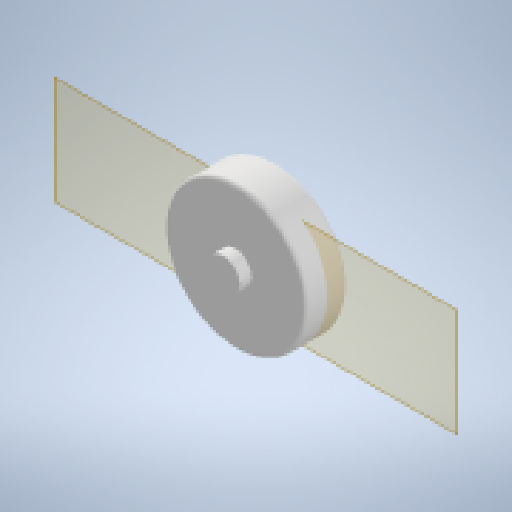
# Autodesk Inventor part: Колесо
Saved by Autodesk Inventor 2024.2 (Build 282272000, 272)
## iProperties
Created: 2025-03-03
Part Number: Колесо
Material: Типовые
Document SubType Name: Modeling
Designer: Timofey
Density: 1 g/cm^3
Appearance: По умолчанию
Mass: 1234.52 g
Surface Area: 769.826 cm^2
Volume: 1234.52 cm^3
Author: Timofey
Autodesk Inventor part; units mm, degrees
ref_plane "YZ Plane" through (0, 0, 0) normal (1, 0, 0) x (0, 1, 0)
ref_plane "XZ Plane" through (0, 0, 0) normal (0, 1, 0) x (-1, 0, 0)
ref_plane "XY Plane" through (0, 0, 0) normal (0, 0, 1) x (1, 0, 0)
ref_plane "РабПлоскость3" through (0.0801, 60, -30) normal (0, 0, 1) x (1, 0, 0)
sketch "Эскиз1" plane through (0.0801, 60, -30) normal (0, 0, 1) x (1, 0, 0)
  line L0 (-0.0801, -60) -> (-90.0801, -60)
  circle A0 centre (-90.0801, -60) radius 87.5
  dimension "d0" = 90
  dimension "d1" = 175
  constraints: 2 end point, 1 centre point, 1 coincident, 1 horizontal
  measures "d0" distance of L0.start L0.end
  measures "d1" diameter of A0
extrude "Выдавливание1" add sketch "Эскиз1" along normal mid plane 50
sketch "Эскиз2" plane through (-90, 0, -5) normal (0, 0, 1) x (1, 0, 0)
  circle A0 centre (0, 0) radius 20
  point P0 (90, 0)
  dimension "d4" = 40
  constraints: 1 centre point
  measures "d4" diameter of A0
extrude "Выдавливание2" add sketch "Эскиз2" along normal blind 15
sketch "Эскиз3" plane through (-90, 0, -55) normal (0, 0, -1) x (-1, 0, 0)
  circle A0 centre (0, 0) radius 20 projected
  circle A1 centre (0, 0) radius 20
  point P0 (-90, 0)
  dimension "d7" = 40
  constraints: 1 centre point, 1 coincident
  measures "d7" diameter of A1
extrude "Выдавливание3" add sketch "Эскиз3" along normal blind 15
fillet "Сопряжение1" radius 5 1 edges at (-177.5, 0, -5)
fillet "Сопряжение2" radius 5 1 edges at (-177.5, 0, -55)
